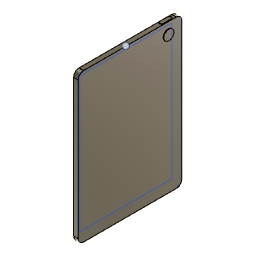
Untitled (Autodesk Fusion 360 design; units mm, degrees)
Autodesk Fusion 360 part; units mm, degrees
sketch "Sketch1" plane through (0, 0, 0) normal (1, 0, 0) x (0, 1, 0)
  line L0 (0, 0) -> (169, 0)
  line L1 (169, 0) -> (169, 242.1233)
  line L2 (169, 242.1233) -> (0, 242.1233)
  line L3 (0, 242.1233) -> (0, 0)
  dimension "d1" = 169
  constraint horizontal L0
  constraint vertical L1
  constraint horizontal L2
  constraint vertical L3
  constraint coincident L0.start L3.end
  measures "d1" distance of L0.start L0.end
extrude "Extrude1" add sketch "Sketch1" along normal blind 7.5
sketch "Sketch2" plane through (0, 0, 0) normal (-1, 0, 0) x (0, -1, 0)
  line L0 (0, 0) -> (0, 242.1233)
  line L1 (0, 242.1233) -> (-169, 242.1233)
  line L2 (-169, 242.1233) -> (-169, 0)
  line L3 (-169, 0) -> (0, 0)
fillet "Fillet1" radius 9 1 edges at (3.75, 0, 242.1233)
fillet "Fillet2" radius 9 1 edges at (3.75, 169, 242.1233)
fillet "Fillet3" radius 9 1 edges at (3.75, 0, 0)
fillet "Fillet4" radius 9 1 edges at (3.75, 169, 0)
sketch "Sketch3" plane through (0, 0, 0) normal (-1, 0, 0) x (0, -1, 0)
  circle A0 centre (-85, 235) radius 5
sketch "Sketch4" plane through (0, 0, 0) normal (-1, 0, 0) x (0, -1, 0)
  circle A0 centre (-84.9515, 235.215) radius 0
sketch "Sketch5" plane through (0, 0, 0) normal (-1, 0, 0) x (0, -1, 0)
  circle A0 centre (-85.1812, 235.1149) radius 3
  dimension "d8" = 6
  measures "d8" diameter of A0
sketch "Sketch6" plane through (0, 0, 0) normal (-1, 0, 0) x (0, -1, 0)
  line L0 (-10, 230) -> (-160, 230)
  line L1 (-160, 230) -> (-160, 10)
  line L2 (-160, 10) -> (-10, 10)
  line L3 (-10, 10) -> (-10, 230)
  constraint horizontal L0
  constraint vertical L1
  constraint horizontal L2
  constraint vertical L3
sketch "Sketch7" plane through (0, 0, 0) normal (-1, 0, 0) x (0, -1, 0)
sketch "Sketch8" plane through (0, 0, 0) normal (-1, 0, 0) x (0, -1, 0)
sketch "Sketch9" plane through (0, 0, 0) normal (-1, 0, 0) x (0, -1, 0)
sketch "Sketch10" plane through (0, 0, 0) normal (-1, 0, 0) x (0, -1, 0)
sketch "Sketch11" plane through (0, 0, 0) normal (0, 0, -1) x (1, 0, 0)
  line L0 (0, -160) -> (7.5, -160)
  line L1 (7.5, -160) -> (7.5, -9)
  line L2 (7.5, -9) -> (0, -9)
  line L3 (0, -9) -> (0, -160)
sketch "Sketch12" plane through (0, 0, 242.1233) normal (0, 0, 1) x (-1, 0, 0)
  line L0 (-7.5, -160) -> (0, -160)
  line L1 (0, -160) -> (0, -9)
  line L2 (0, -9) -> (-7.5, -9)
  line L3 (-7.5, -9) -> (-7.5, -160)
  line L4 (-1, -155) -> (-7, -155)
  line L5 (-7, -155) -> (-7, -137)
  line L6 (-7, -137) -> (-1, -137)
  line L7 (-1, -137) -> (-1, -155)
  constraint horizontal L4
  constraint vertical L5
  constraint horizontal L6
  constraint vertical L7
extrude "Extrude2" add sketch "Sketch12" along normal blind 1 contours L4 L5 L6 L7
fillet "Fillet5" radius 2 1 edges at (1, 155, 242.6233)
fillet "Fillet6" radius 2 1 edges at (7, 155, 242.6233)
fillet "Fillet7" radius 2 1 edges at (1, 137, 242.6233)
fillet "Fillet8" radius 2 1 edges at (7, 137, 242.6233)
sketch "Sketch13" plane through (7.5, 0, 0) normal (1, 0, 0) x (0, 1, 0)
  arc A0 (160, 0) -> (169, 9) centre (160, 9) ccw
  line L0 (169, 9) -> (169, 233.1233)
  arc A1 (169, 233.1233) -> (160, 242.1233) centre (160, 233.1233) ccw
  line L1 (160, 242.1233) -> (9, 242.1233)
  arc A2 (9, 242.1233) -> (0, 233.1233) centre (9, 233.1233) ccw
  line L2 (0, 233.1233) -> (0, 9)
  arc A3 (0, 9) -> (9, 0) centre (9, 9) ccw
  line L3 (9, 0) -> (160, 0)
  circle A4 centre (146.9534, 223.7975) radius 8.2997
  circle A5 centre (147.3608, 209.8046) radius 2.0283
  dimension "d15" = 16.5995
  measures "d15" diameter of A4
extrude "Extrude3" add sketch "Sketch13" along normal blind 1 contours A4
